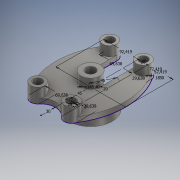
# Autodesk Inventor part: Вилка
Saved by Autodesk Inventor 2018 (Build 220112000, 112)
## iProperties
Created: 2020-04-13
Part Number: Вилка
Material: Сталь, мягкая
Document SubType Name: ЛистМат
Designer: Alena Oparina
Density: 7.85 g/cm^3
Appearance: С умеренной полировкой
Sheet Metal Rule: По умолчанию_мм
Author: Alena Oparina
Autodesk Inventor part; units mm, degrees
ref_plane "YZ Plane" through (0, 0, 0) normal (1, 0, 0) x (0, 1, 0)
ref_plane "XZ Plane" through (0, 0, 0) normal (0, 1, 0) x (-1, 0, 0)
ref_plane "XY Plane" through (0, 0, 0) normal (0, 0, 1) x (1, 0, 0)
sketch "Эскиз1" plane through (0, 0, 0) normal (0, 0, 1) x (1, 0, 0)
  circle A0 centre (0, 0) radius 20
  circle A1 centre (0, 0) radius 10
  circle A2 centre (-35, 75) radius 15
  circle A3 centre (-35, 75) radius 9
  circle A4 centre (35, 75) radius 15
  circle A5 centre (35, 75) radius 9
  circle A6 centre (-35, -75) radius 15
  circle A7 centre (-35, -75) radius 9
  circle A8 centre (35, -75) radius 15
  circle A9 centre (35, -75) radius 9
  arc A10 (23, -84) -> (-23, -84) centre (0, -103.2614) ccw
  arc A11 (-20, 40.3113) -> (20, 40.3113) centre (0, 0) ccw
  line L0 (-20, 40.3113) -> (-20, 0)
  line L1 (-20, 40.3113) -> (-20, 75)
  line L2 (20, 40.3113) -> (20, 0)
  line L3 (20, 40.3113) -> (20, 75)
  arc A12 (-49.6377, 78.2768) -> (-49.6377, -78.2768) centre (72.4186, 0) ccw
  arc A13 (49.6377, -78.2768) -> (49.6377, 78.2768) centre (-72.4186, 0) ccw
  dimension "d75" = 145
  dimension "d76" = 30
  dimension "d77" = 18
  dimension "d78" = 45
  dimension "d79" = 40
  dimension "d80" = 20
  dimension "d81" = 30
  dimension "d82" = 20
  dimension "d83" = 52.4186
  dimension "d84" = 29.6377
  dimension "d85" = 29.6377
  dimension "d86" = 3
  dimension "d87" = 20
  dimension "d88" = 43
  dimension "d89" = 69.6377
  dimension "d90" = 69.6377
  dimension "d91" = 92.4186
  dimension "d92" = 72.4186
  dimension "d93" = 45
  constraints: 18 point on circle, 14 centre point, 8 end point, 7 equal radius, 6 coincident, 6 tangent, 3 vertical, 1 point on line
  measures "d75" radius of A12
  measures "d76" diameter of A4
  measures "d77" diameter of A5
  measures "d78" radius of A11
  measures "d79" diameter of A0
  measures "d80" diameter of A1
  measures "d81" radius of A10
  measures "d82" distance from line of point (0, 0) L2
  measures "d83" distance from line of A12.centre L2
  measures "d84" distance from line of A4.end L2
  measures "d85" distance from line of A8.end L2
  measures "d86" distance from line of A8.start L2
  measures "d87" distance from line of A10.centre L2
  measures "d88" distance from line of A6.start L2
  measures "d89" distance from line of A2.end L2
  measures "d90" distance from line of A6.end L2
  measures "d91" distance from line of A13.centre L2
  measures "d92" distance of point (0, 0) A12.centre
  measures "d93" distance of point (0, 0) L2.start
extrude "Выдавливание1" add sketch "Эскиз1" along normal blind 10 contours L3 A4 A13 A8 A10 A6 A12 A2 L1 A11
extrude "Выдавливание2" add sketch "Эскиз1" along normal blind 30 contours A4 | A2 | A8 | A6
extrude "Выдавливание3" add sketch "Эскиз1" along normal blind 30 contours A0
extrude "Выдавливание4" add sketch "Эскиз1" along normal blind 10 contours L2 A11 L0 A0
extrude "Выдавливание5" add sketch "Эскиз1" against normal blind 40 contours L2 A11 L0 A0
